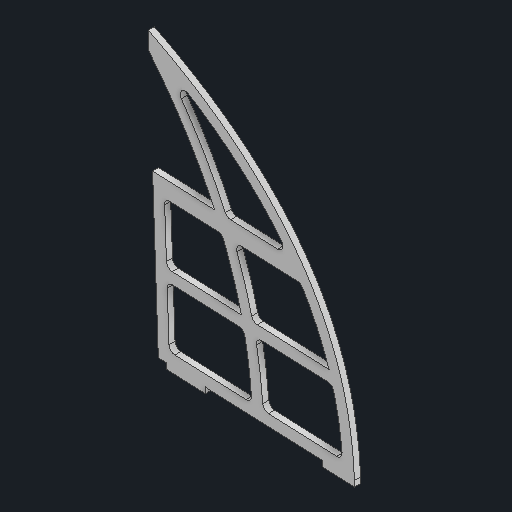
# Autodesk Inventor part: sponson_spanner_side
Saved by Autodesk Inventor 2022.2 (Build 262287010, 287A)
## iProperties
Created: 2022-03-22
Part Number: sponson_spanner_side
Material: Generic
Document SubType Name: Modeling
Designer: kardo
Density: 1 g/cm^3
Appearance: Default
Author: kardo
Autodesk Inventor part; units mm, degrees
ref_plane "YZ Plane" through (0, 0, 0) normal (1, 0, 0) x (0, 1, 0)
ref_plane "XZ Plane" through (0, 0, 0) normal (0, 1, 0) x (-1, 0, 0)
ref_plane "XY Plane" through (0, 0, 0) normal (0, 0, 1) x (1, 0, 0)
derived "surface_body.ipt"
sketch "sk_rail_sponson_side" plane through (81.12, 237, 36.448) normal (0.0378267, 0.0348745, -0.9986756) x (0.3011979, -0.9533106, -0.0218819)
  line L0 (248.6073, 0) -> (121.4703, -40.1899)
  spline S0 degree 2 poles (121.4703, -40.1899) (54.6944, -61.2988) (0, 0) knots 0 0 0 1 1 1
  point P0 (202.299, 150.0824)
ref_plane "plane_tunnel_right" through (81.12, 0, 0) normal (1, 0, 0) x (0, 1, 0)
ref_plane "plane_sponson_side" through (81.12, 237, 36.448) normal (0.0378267, 0.0348745, -0.9986756) x (0.3011979, -0.9533106, -0.0218819)
sketch "sk_rail_sponson_tunnel" plane through (81.12, 0, 0) normal (1, 0, 0) x (0, 1, 0)
  line L0 (0, 0) -> (135.09, 9.4464)
  line L1 (125.2485, 150.1861) -> (152.4642, -239.0164) construction
  spline S0 degree 2 poles (135.09, 9.4464) (188.144, 13.1563) (237, 36.448) knots 0 0 0 1 1 1
sketch "sk_rail_sponson_bottom" plane through (126.048, 0, 0) normal (0.4037383, -0.0638184, 0.9126459) x (-0.1841621, 0.9714748, 0.1494022)
  line L0 (132.6478, -27.2597) -> (0, 0)
  line L1 (373.4222, -76.7399) -> (-490.1731, 100.7327) construction
  line L2 (179.8623, 202.4893) -> (98.6127, -192.8771) construction
  spline S0 degree 2 poles (132.6478, -27.2597) (191.4823, -39.3504) (243.959, 0) knots 0 0 0 1 1 1
  point P0 (23.2133, 112.9576)
sketch "sk_rail_top_tunnel" plane through (81.12, 0, 0) normal (1, 0, 0) x (0, 1, 0)
  line L0 (237, 107.6209) -> (237, -224.5198) construction
  line L1 (0, 107.6209) -> (0, -224.5198) construction
  line L2 (-363, 107.6209) -> (-363, -224.5198) construction
  line L3 (-363, 0) -> (0, 0) construction
  line L4 (-181.5, 48.8998) -> (-181.5, 0) construction
  line L5 (0, 52.89) -> (52.14, 52.89) construction
  line L6 (52.14, 52.89) -> (75.84, 48.2838) construction
  line L7 (75.84, 48.2838) -> (94.8, 37.536) construction
  line L8 (94.8, 107.6209) -> (94.8, -224.5198) construction
  line L9 (0, 52.89) -> (237, 52.89) construction
  line L10 (-488.1035, 0) -> (361.1125, 0) construction
  spline S0 degree 3 poles (0, 52.89) (86.3106, 52.89) (181.3207, 49.5034) (237, 36.448) knots 0 0 0 0 1 1 1 1
  spline S1 degree 3 poles (0, 52.89) (52.14, 52.89) (75.84, 48.2838) (94.8, 37.536) knots 1 1 1 1 2 2 2 2
  spline S2 degree 4 poles (-363, 37.4293) (-272.3626, 45.1427) (-181.5879, 49.7528) (-90.8131, 52.89) (0, 52.89) knots 0 0 0 0 0 1 1 1 1 1
  point P0 (142.2, 48.7795)
  point P1 (94.8, 28.832)
  point P2 (-242.0001, 45.8501)
  point P3 (-120.9999, 51.0063)
sketch "sk_section_sponson_break" plane through (0, 135.09, 9.4464) normal (0, 0.9975641, 0.0697565) x (-1, 0, 0)
  line L0 (-276.9076, -66.575) -> (63.0269, 83.4396) construction
  line L1 (-81.12, -263.4566) -> (-81.12, 154.4936) construction
  arc A0 (-81.12, 40.0762) -> (-156, 26.279) centre (-76.0371, -197.602) ccw construction
  arc A1 (-54.6, 54.2675) -> (-156, 30.9325) centre (-53.2768, -183.4615) ccw construction
  spline S0 degree 2 poles (-54.6, 54.2675) (-107.2974, 54.2675) (-156, 30.9325) knots 0 0 0 1 1 1
  spline S1 degree 2 poles (-156, 26.279) (-119.9166, 39.1668) (-81.12, 40.0762) knots 0 0 0 1 1 1
  point P0 (0, 0)
ref_plane "plane_sponson_break" through (0, 135.09, 9.4464) normal (0, 0.9975641, 0.0697565) x (-1, 0, 0)
derived "parameters_frame.ipt"
derived "stencil_frame.ipt"
sketch "sk_joint_locations" plane through (81.12, 0, 0) normal (1, 0, 0) x (0, 1, 0)
  line L0 (0, 0) -> (135.09, 9.4464) construction
  line L1 (30.81, 28.832) -> (94.8, 28.832) construction
  arc A0 (30.81, 28.832) -> (9.48, 28.4869) centre (30.81, -630.4631) ccw construction
  line L2 (-254.1001, 19.9549) -> (9.48, 28.4869) construction
  line L3 (-363, 18.496) -> (-275.8801, 19.4795) construction
  arc A1 (-275.8801, 19.4795) -> (-254.1001, 19.9549) centre (-287.5515, 1053.3708) ccw construction
  line L4 (25.1322, 1581.9163) -> (267.6663, -1886.4825) construction
  line L5 (-242.0001, 1541.8302) -> (-242.0001, -1877.3857) construction
  line L6 (-120.9999, 1541.8302) -> (-120.9999, -1877.3857) construction
  line L7 (-363, 1541.8302) -> (-363, -1877.3857) construction
  line L8 (0, 1541.8302) -> (0, -1877.3857) construction
  line L9 (450.0665, 43.8884) -> (-613.9211, 6.7332) construction
  line L10 (-677.4829, -27.4989) -> (501.7293, 54.9597) construction
  line L11 (187.7215, 30.7247) -> (187.4423, 38.7198) construction
  line L12 (195.4031, 37.5588) -> (195.9625, 29.5588) construction
  line L13 (0, 3.808) -> (134.9306, 11.7256) construction
  line L14 (-242.0001, 45.8501) -> (-242.0001, 20.3465) construction
  line L15 (-363, 37.4293) -> (-363, 18.496) construction
  line L16 (-120.9999, 51.0063) -> (-120.9999, 24.2633) construction
  line L17 (0, 52.89) -> (0, 28.18) construction
  line L18 (132.2944, 49.425) -> (132.8217, 41.8851) construction
  line L19 (133.3489, 34.3453) -> (132.8217, 41.8851) construction
  line L20 (133.3489, 34.3453) -> (133.8761, 26.8054) construction
  line L21 (133.8761, 26.8054) -> (134.4034, 19.2655) construction
  line L22 (134.4034, 19.2655) -> (134.9306, 11.7256) construction
  line L23 (0, 3.808) -> (0, 0) construction
  line L24 (94.8, 37.536) -> (94.8, 28.832) construction
  line L25 (94.8, 35.548) -> (94.8, 30.82) construction
  spline S0 degree 4 poles (-363, 37.4293) (-272.3626, 45.1427) (-181.5879, 49.7528) (-90.8131, 52.89) (0, 52.89) knots 0 0 0 0 0 1 1 1 1 1
  spline S1 degree 3 poles (0, 52.89) (86.3106, 52.89) (181.3207, 49.5034) (237, 36.448) knots 0 0 0 0 1 1 1 1
  spline S2 degree 2 poles (135.09, 9.4464) (188.144, 13.1563) (237, 36.448) knots 0 0 0 1 1 1
  point P0 (187.5819, 34.7223)
  point P1 (195.6828, 33.5588)
  point P2 (134.9575, 11.3411)
  point P3 (-363, 27.9627)
  point P4 (-242.0001, 33.0983)
  point P5 (-120.9999, 37.6348)
  point P6 (0, 40.535)
  point P7 (94.8, 33.184)
sketch "sk_spanner_joints_locations" plane through (0, 135.09, 9.4464) normal (0, 0.9975641, 0.0697565) x (-1, 0, 0)
  line L0 (266.3539, 10.2816) -> (-340.3092, 33.2601) construction
  line L1 (-958.4738, -367.3533) -> (724.0529, 375.1534) construction
  line L2 (-86.9102, 23.6621) -> (-85.7837, 17.7688) construction
  line L3 (-86.9102, 23.6621) -> (-73.574, 23.157) construction
  line L4 (-85.7837, 17.7688) -> (-73.574, 23.157) construction
  point P0 (0, 0)
  point P1 (-126.048, 0)
  point P2 (-156, 26.279)
  point P3 (-142.182, 25.7557)
  point P4 (-100.7281, 24.1855)
  point P5 (-95.8498, 13.3266)
  point P6 (-115.9819, 4.4422)
ref_plane "plane_stringer_outer" through (84.12, 0, 0) normal (1, 0, 0) x (0, 1, 0)
sketch "sk_corner_offset" plane through (0, 135.09, 9.4464) normal (0, 0.9975641, 0.0697565) x (-1, 0, 0)
  spline S0 degree 2 poles (-156, 26.279) (-119.9166, 39.1668) (-81.12, 40.0762) knots 0 0 0 1 1 1 construction
  line L0 (-156, 26.279) -> (-126.048, 0) construction
  line L1 (-153.6672, 25.8287) -> (-125.2566, 0.902) construction
  line L2 (-125.2566, 0.902) -> (-126.048, 0) construction
  spline S1 degree 5 poles (-153.6672, 25.8287) (-139.6799, 30.69) (-125.3161, 34.4683) (-110.6738, 37.0828) (-95.8958, 38.5294) (-81.0919, 38.8766) knots 0 0 0 0 0 0 1 1 1 1 1 1 construction
  point P0 (0, 0)
  dimension "d9" = 1.2
  dimension "d10" = 1.2
  constraints: 6 end point, 1 coincident, 1 parallel, 1 perpendicular, 3 other
  measures "d10" distance between parallel lines of L1 L0
sketch "sk_tip_offset" plane through (81.12, 0, 0) normal (1, 0, 0) x (0, 1, 0)
  spline S0 degree 3 poles (0, 52.89) (86.3106, 52.89) (181.3207, 49.5034) (237, 36.448) knots 0 0 0 0 1 1 1 1 construction
  spline S1 degree 2 poles (135.09, 9.4464) (188.144, 13.1563) (237, 36.448) knots 0 0 0 1 1 1 construction
  spline S2 degree 5 poles (0, 51.69) (13.1181, 51.69) (26.2363, 51.6248) (39.354, 51.4874) (65.3463, 51.0551) (91.3298, 50.254) (104.1978, 49.754) (128.8047, 48.5691) (153.3792, 46.8416) (165.0971, 45.8705) (185.8514, 43.8357) (206.5158, 41.0381) (215.5021, 39.6373) (224.4562, 38.0172) (233.3343, 36.0522) knots 0 0 0 0 0 0 0.280033 0.280033 0.280033 0.55492 0.55492 0.55492 0.805891 0.805891 0.805891 1 1 1 1 1 1 construction
  spline S3 degree 5 poles (135.0063, 10.6435) (155.3816, 12.0688) (175.6301, 15.3217) (195.5215, 20.4957) (214.7957, 27.4783) (233.3343, 36.0523) knots 0 0 0 0 0 0 1 1 1 1 1 1 construction
  point P0 (0, 0)
  dimension "d7" = 1.2
  dimension "d8" = 1.2
  constraints: 1 coincident, 6 other
sketch "sk_sponson_spanner_side_base" plane through (81.12, 237, 36.448) normal (0.0378267, 0.0348745, -0.9986756) x (0.3011979, -0.9533106, -0.0218819)
  spline S0 degree 2 poles (121.4703, -40.1899) (54.6944, -61.2988) (0, 0) knots 0 0 0 1 1 1 construction
  line L0 (100.5437, 25.7064) -> (99.6986, 28.3676)
  line L1 (104.729, 12.5272) -> (117.285, -27.0106)
  line L2 (117.285, -27.0106) -> (119.1912, -26.4053)
  line L3 (119.1912, -26.4053) -> (122.6666, -37.3491)
  line L4 (104.729, 12.5272) -> (106.6352, 13.1325)
  line L5 (106.6352, 13.1325) -> (102.4499, 26.3118)
  line L6 (102.4499, 26.3118) -> (100.5437, 25.7064)
  line L7 (729.616, 227.494) -> (-188.5213, -62.743) projected
  line L8 (122.6666, -37.3491) -> (120.7476, -37.9557)
  line L9 (248.6073, 0) -> (121.4703, -40.1899) construction
  spline S1 degree 2 poles (3.5032, 1.118) (56.2109, -58.3567) (120.7476, -37.9557) knots 0 0 0 1 1 1
  point P0 (202.299, 150.0824)
  point P1 (47.1486, 14.9044)
  point P2 (99.6986, 28.3676)
  point P3 (2.2186, -2.4472)
  point P4 (5.7186, -1.3409)
  dimension "d3" = 2
  constraints: 16 end point, 4 parallel, 2 collinear, 2 perpendicular, 1 point on line, 3 other
  measures "d3" distance between parallel lines of L5 L1
extrude "thicken" add sketch "sk_sponson_spanner_side_base" along normal blind 2
sketch "sk_cut_weight" plane through (81.12, 237, 36.448) normal (0.0378267, 0.0348745, -0.9986756) x (0.3011979, -0.9533106, -0.0218819)
  line L0 (100.5437, 25.7064) -> (99.6986, 28.3676) construction
  line L1 (104.729, 12.5272) -> (117.285, -27.0106) construction
  spline S0 degree 2 poles (3.5032, 1.118) (56.2109, -58.3567) (120.7476, -37.9557) knots 0 0 0 1 1 1 construction
  line L2 (47.1486, 14.9044) -> (63.0582, -35.4243) construction
  line L3 (53.0731, 9.4335) -> (59.225, -10.0275)
  line L4 (46.1465, 11.439) -> (52.7747, -9.5288)
  line L5 (46.1465, 11.439) -> (11.7093, 0.5529)
  line L6 (53.0731, 9.4335) -> (97.0953, 23.3496)
  line L7 (97.0953, 23.3496) -> (105.9681, -4.5902)
  line L8 (60.5108, -14.0951) -> (67.6472, -36.6702)
  line L9 (54.0839, -13.6702) -> (60.7289, -34.6911)
  line L10 (107.1792, -8.4039) -> (115.7149, -35.282)
  line L11 (75.0842, 16.3916) -> (92.6183, -39.0759) construction
  line L12 (81.1626, -9.4722) -> (73.1772, 15.7887)
  line L13 (76.9912, 16.9944) -> (85.2042, -8.9868)
  line L14 (86.4274, -12.8562) -> (94.6797, -38.9616)
  line L15 (82.3924, -13.3625) -> (90.5425, -39.1446)
  line L16 (729.616, 227.494) -> (-188.5213, -62.743) construction
  spline S1 degree 2 poles (111.007, -7.2417) (59.1117, -23.7221) (5.7186, -1.3409) knots 0 0 0 1 1 1
  spline S2 degree 5 poles (14.5666, -4.7866) (19.5131, -9.7013) (24.7087, -14.3654) (30.1742, -18.7236) (42.5042, -27.2377) (56.0994, -33.5638) (63.6939, -36.1796) (78.7315, -39.4615) (94.1061, -39.4415) (101.4439, -38.6742) (108.6565, -37.2559) (115.7149, -35.282) knots 0 0 0 0 0 0 0.313173 0.313173 0.313173 0.670823 0.670823 0.670823 1 1 1 1 1 1
  spline S3 degree 5 poles (105.9681, -4.5902) (96.8325, -7.2297) (87.4895, -9.1503) (77.9951, -10.2693) (58.7004, -10.8272) (39.5903, -8.0796) (30.0745, -5.8786) (20.7729, -2.9698) (11.7093, 0.5529) knots 0 0 0 0 0 0 0.494415 0.494415 0.494415 1 1 1 1 1 1
  point P0 (202.299, 150.0824)
  dimension "d11" = 4
  dimension "d20" = 4
  dimension "d14" = 2
  dimension "d15" = 4
  dimension "d16" = 4
  dimension "d19" = 4
  dimension "d21" = 4
  constraints: 28 end point, 6 collinear, 5 parallel, 3 point on line, 2 midpoint, 2 perpendicular, 28 other
  measures "d14" distance between parallel lines of L2 L4
  measures "d15" distance between parallel lines of L2 L3
  measures "d16" distance between parallel lines of L1 L7
  measures "d19" distance between parallel lines of L13 L12
  measures "d21" distance between parallel lines of L16 L6
extrude "cut_weight" cut sketch "sk_cut_weight" along normal through all both and the other way through all contours L6 L12 S3 L3 | L6 L7 S3 L13 | L4 S3 L5 | S1 L15 S2 L8 | L9 S2 S1 | S1 L10 S2 L14
fillet "rounding" radius 2 17 edges at (88.155, 137.4687, 32.2374) (121.4473, 137.3807, 33.4954) (118.7061, 162.4977, 34.2686) (88.155, 162.5381, 33.1129) (110.4729, 189.5768, 34.9024) (88.155, 158.5405, 32.9733) (88.155, 183.61, 33.8487) (112.8135, 183.5774, 34.7816) (90.106, 224.5842, 35.3535) (119.4392, 158.4992, 34.1568) (108.5506, 183.583, 34.6203) (136.4728, 183.5461, 35.6766) (115.3838, 158.5046, 34.0034) (146.7982, 158.4631, 35.1918) (132.5032, 189.5477, 35.7358) (149.6279, 137.3062, 34.5602) (117.4488, 137.3913, 33.3443)
equation "\"d9\" = shell_thickness"
equation "\"d10\" = shell_thickness"
equation "\"d7\" = shell_thickness"
equation "\"d8\" = shell_thickness"
equation "\"d3\" = bulkhead_thickness"
equation "\"d5\" = bulkhead_thickness"
equation "\"d11\" = bulkhead_inset"
equation "\"d20\" = bulkhead_inset"
equation "\"d14\" = bulkhead_thickness"
equation "\"d15\" = 2 * bulkhead_thickness"
equation "\"d16\" = bulkhead_inset"
equation "\"d19\" = bulkhead_inset"
equation "\"d21\" = bulkhead_inset"
equation "\"d25\" = 0.5 * bulkhead_inset"
equation "\"d4\" = stringer_thickness"
equation "\"shell_thickness\" = 1.2"
equation "\"bulkhead_thickness\" = 2"
equation "\"bulkhead_inset\" = 4"
equation "\"stringer_thickness\" = 3"
body "Solid1"
